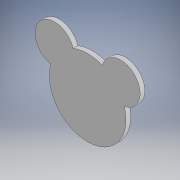
# Autodesk Inventor part: BackPiece
Saved by Autodesk Inventor 2019 (Build 230136000, 136)
## iProperties
Created: 2020-02-13
Part Number: BackPiece
Material: Generic
Document SubType Name: Modeling
Designer: student
Density: 1 g/cm^3
Appearance: Default
Author: student
Autodesk Inventor part; units mm, degrees
ref_plane "YZ Plane" through (0, 0, 0) normal (1, 0, 0) x (0, 1, 0)
ref_plane "XZ Plane" through (0, 0, 0) normal (0, 1, 0) x (-1, 0, 0)
ref_plane "XY Plane" through (0, 0, 0) normal (0, 0, 1) x (1, 0, 0)
sketch "Sketch1" plane through (0, 0, 0) normal (0, 0, 1) x (1, 0, 0)
  arc A0 (-14.4595, 35.2496) -> (-36.5756, 10.6694) centre (-32.9209, 29.6206) ccw
  arc A1 (36.5756, 10.6694) -> (14.4595, 35.2496) centre (32.9209, 29.6206) ccw
  arc A2 (-36.5756, 10.6694) -> (36.5756, 10.6694) centre (0, 0) ccw
  arc A3 (14.4595, 35.2496) -> (-14.4595, 35.2496) centre (0, 0) ccw
  constraints: 8 point on circle, 4 centre point, 1 coincident
extrude "Extrusion1" add sketch "Sketch1" along normal blind 4.699
sketch "Sketch2" plane through (0, 0, 0) normal (0, 0, -1) x (-1, 0, 0)
  arc A0 (36.5756, 10.6694) -> (14.4595, 35.2496) centre (32.9209, 29.6206) ccw projected
  arc A1 (14.4595, 35.2496) -> (-14.4595, 35.2496) centre (0, 0) ccw projected
  arc A2 (-14.4595, 35.2496) -> (-36.5756, 10.6694) centre (-32.9209, 29.6206) ccw projected
  arc A3 (-36.5756, 10.6694) -> (36.5756, 10.6694) centre (0, 0) ccw projected
  arc A4 (-36.5756, 10.6694) -> (36.5756, 10.6694) centre (0, 0) ccw projected
  line L0 (-21.0606, -31.75) -> (21.0606, -31.75)
  point P0 (0, -38.1)
  dimension "d4" = 6.35
  constraints: 3 point on circle, 2 end point, 1 horizontal
  measures "d4" distance from line of L0 point (0, -38.1)
extrude "Extrusion2" cut sketch "Sketch2" against normal blind 25.4 contours A3 L0
fillet "Fillet1" radius 3.175 2 edges at (21.0606, -31.75, 2.3495) (-21.0606, -31.75, 2.3495)
body "Solid1"
